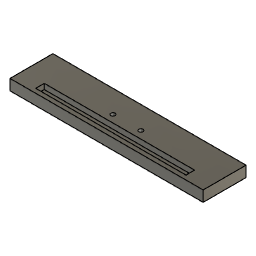
AttacheDown v4 (Autodesk Fusion 360 design; units mm, degrees)
Autodesk Fusion 360 part; units mm, degrees
sketch "Esquisse1" plane through (0, 0, 0) normal (0, 0, 1) x (1, 0, 0)
  line L0 (0, 0) -> (90, 0)
  line L1 (90, 0) -> (90, 20)
  line L2 (90, 20) -> (0, 20)
  line L3 (0, 20) -> (0, 0)
  circle A0 centre (38.5, 9.5) radius 1
  circle A1 centre (51.5, 9.5) radius 1
  dimension "d1" = 90
  dimension "d2" = 20
  dimension "d3" = 2
  dimension "d4" = 2
  dimension "d5" = 13
  dimension "d6" = 9.5
  dimension "d7" = 9.5
  dimension "d8" = 38.5
  constraint horizontal L0
  constraint vertical L1
  constraint horizontal L2
  constraint vertical L3
  constraint coincident L0.start L3.end
  measures "d1" distance of L1.end L2.end
  measures "d2" distance of L0.end L1.end
  measures "d3" diameter of A0
  measures "d4" diameter of A1
  measures "d5" distance of A0.centre A1.centre
  measures "d6" distance of L0 A1.centre
  measures "d7" distance of L0 A0.centre
  measures "d8" distance of L1 A1.centre
extrude "Extrusion1" add sketch "Esquisse1" along normal blind 5
sketch "Esquisse2" plane through (0, 0, 5) normal (0, 0, 1) x (-1, 0, 0)
  circle A0 centre (-38.5, -9.5) radius 1
  circle A1 centre (-51.5, -9.5) radius 1
  line L0 (0, -20) -> (0, 0)
  line L1 (0, 0) -> (-90, 0)
  line L2 (-90, 0) -> (-90, -20)
  line L3 (-90, -20) -> (0, -20)
  line L4 (-10, -6) -> (-80, -6)
  line L5 (-80, -6) -> (-80, -2)
  line L6 (-80, -2) -> (-10, -2)
  line L7 (-10, -2) -> (-10, -6)
  dimension "d11" = 2
  dimension "d12" = 4
  dimension "d13" = 10
  dimension "d14" = 70
  constraint horizontal L4
  constraint vertical L5
  constraint horizontal L6
  constraint vertical L7
  measures "d11" distance of L1 L6
  measures "d12" distance of L4.start L6.end
  measures "d13" distance of L0 L7
  measures "d14" distance of L5.end L6.end
extrude "Extrusion2" cut sketch "Esquisse2" against normal blind 2.5 contours L4 L5 L6 L7
